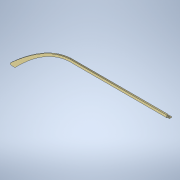
# Autodesk Inventor part: brat bun ochelari
Saved by Autodesk Inventor 2020 (Build 240168000, 168)
## iProperties
Created: 2019-12-24
Part Number: brat bun ochelari
Material: Iron, Cast
Document SubType Name: Modeling
Designer: Bianca
Density: 7.15 g/cm^3
Appearance: Iron Gray
Mass: 2.67895 g
Surface Area: 9.83694 cm^2
Volume: 0.374679 cm^3
Author: Bianca
Autodesk Inventor part; units mm, degrees
ref_plane "YZ Plane" through (0, 0, 0) normal (1, 0, 0) x (0, 1, 0)
ref_plane "XZ Plane" through (0, 0, 0) normal (0, 1, 0) x (-1, 0, 0)
ref_plane "XY Plane" through (0, 0, 0) normal (0, 0, 1) x (1, 0, 0)
sketch "Sketch1" plane through (0, 0, 0) normal (0, 0, 1) x (1, 0, 0)
  line L0 (0, 0) -> (-80, 0)
  line L1 (-80, 2) -> (0, 2)
  line L2 (0, 2) -> (0, 0)
  line L3 (-80, 2) -> (-84.2329, 2)
  line L4 (-133.3122, -28) -> (-131.553, -28)
  spline S0 degree 2 poles (-80, 0) (-102.6249, 1.8185) (-131.553, -28) knots 0 0 0 1 1 1
  spline S1 degree 2 poles (-80, 2) (-102.2926, 3.4342) (-135, -26) knots 0 0 0 1 1 1
  spline S2 degree 2 poles (-135, -26) (-137.4492, -28.2041) (-131.553, -28) knots 0 0 0 1 1 1
  line L5 (0, 1.35) -> (0, 1)
  line L6 (0, 0.65) -> (0, 1)
  point P0 (-99.9996, -4.0002)
  point P1 (-100, -1)
  point P2 (-100, -2)
  dimension "d1" = 2
  constraints: 14 end point, 2 horizontal, 1 midpoint, 1 parallel, 13 other
  measures "d1" distance of L0.end L1.start
extrude "Extrusion1" add sketch "Sketch1" along normal blind 1.2 contours L0 S0 L4 S2 S1 L3 L1 L2
sketch "Sketch2" plane through (0, 0, 0) normal (1, 0, 0) x (0, 0, -1)
  line L0 (-1.2, 0) -> (-1.2, 2) projected
  line L1 (0, 0) -> (0, 2) projected
  line L2 (0, 2) -> (-1.2, 2) projected
  line L3 (0.4, 0.85) -> (-1.6, 0.85)
  line L4 (-1.6, 0.85) -> (-1.6, 1.35)
  line L5 (-1.6, 1.35) -> (0.4, 1.35)
  line L6 (0.4, 1.35) -> (0.4, 0.85)
  line L7 (0.4, 0.85) -> (-1.6, 1.35) construction
  line L8 (-1.6, 0.85) -> (0.4, 1.35) construction
  point P0 (-0.6, 1.1)
  dimension "d12" = 2
  dimension "d13" = 0.5
  constraints: 12 end point, 2 midpoint, 2 parallel, 1 horizontal, 1 perpendicular
  measures "d12" distance of L4.end L5.end
  measures "d13" distance of L3.end L4.end
extrude "Extrusion2" add sketch "Sketch2" along normal blind 2.5 contours L3 L4 L5 L0 | L0 L5 L1 L3 | L1 L5 L6 L3
sketch "Sketch3" plane through (0, 1.35, 0) normal (0, 1, 0) x (1, 0, 0)
  line L0 (0, 0) -> (0, -1.2) projected
  line L1 (0, 0.4) -> (2.5, 0.4) projected
  point P0 (1.25, -0.6)
hole "Hole1" at (1.25, 1.35, 0.6) direction (0, -1, 0) diameter 1.25 depth 0.7
fillet "Fillet1" radius 0.3 4 edges at (0, 1.675, 1.2) (0, 1.675, 0) (0, 0.425, 1.2) (0, 0.425, 0)
body "Solid1"
